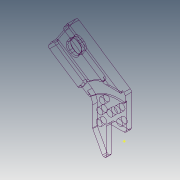
# Autodesk Inventor part: J005046
Saved by Autodesk Inventor 2015 SP1 (Build 190203100, 203)
## iProperties
Created: 2014-10-29
Material: STAINLESS STEEL, 316L
Vendor: HHMI: JFRC - ID&F
Document SubType Name: Sheet Metal
Designer: arnoldj
Density: 8 g/cm^3
Sheet Metal Rule: Default
Description: MBS INLINE REF TAB
Mass: 3.02517 g
Surface Area: 6.77077 cm^2
Volume: 0.378146 cm^3
Project: P-201804
Appearance: Pink
Part Number: J005046
RuleStatus: InUse
AfterDocSave0: file://Part Number Cleaner
DESIGN DEPARTMENT: HHMI: JRC - ID&F
SPECIAL FINISH: NONE
LAB/DEPT: SVOBODA (LAB)
REQUESTING SCIENTIST: SOFRONIEW, NICK
SURFACE ROUGHNESS: 63 Ra
Thickness: 0.050 in
ALTERED ITEM PART NUMBER: N/A
ALTERED ITEM VENDOR: N/A
ALTERED ITEM DESCRIPTION: N/A
Revision Number: A
Autodesk Inventor part; units mm, degrees
note: some values were not read from the file. Chosen so that the rebuilt part matches the saved one: edges of "Fillet8".
ref_plane "YZ Plane" through (0, 0, 0) normal (1, 0, 0) x (0, 1, 0)
sketch "Sketch1" plane through (0, 0, 0) normal (0, 0, 1) x (1, 0, 0)
  line L0 (-4.699, -1.143) -> (-4.699, 6.1251)
  line L1 (4.699, 2.286) -> (4.699, 11.9364)
  line L2 (-4.699, -1.143) -> (-4.699, -1.143) construction
  line L3 (-4.699, -1.143) -> (-1.905, -6.35) construction
  line L4 (-0.889, -6.35) -> (-0.889, 2.286)
  line L5 (4.699, 2.286) -> (-0.889, 2.286)
  line L6 (-0.889, -6.35) -> (-1.905, -6.35)
  line L7 (-1.905, -6.35) -> (-4.699, -1.143)
  line L8 (-4.699, 6.1251) -> (-15.7683, 13.4517)
  line L9 (-15.7683, 13.4517) -> (-10.2307, 21.8181)
  line L10 (-10.2307, 21.8181) -> (4.699, 11.9364)
  line L11 (-15.7683, 13.4517) -> (-28.0607, 13.4517) construction
  line L12 (-12.9995, 17.6349) -> (0, 9.0307) construction
  line L13 (-9.5394, 13.0603) -> (-7.4366, 16.2374)
  line L14 (-7.4366, 16.2374) -> (-10.1053, 18.0038)
  line L15 (-10.1053, 18.0038) -> (-12.2082, 14.8267)
  line L16 (-12.2082, 14.8267) -> (-9.5394, 13.0603)
  line L17 (-9.5394, 13.0603) -> (-10.1053, 18.0038) construction
  line L18 (-7.4366, 16.2374) -> (-12.2082, 14.8267) construction
  point P0 (0, 0)
  point P1 (0, 0)
  point P2 (0, 0)
  point P3 (0, 0)
  point P4 (2.611, -1.214)
  point P5 (-9.8224, 15.532)
  dimension "d102" = 1.016
  dimension "d161" = 123.5
  dimension "d162" = 10.033
  dimension "d168" = 8.636
  dimension "d170" = 5.207
  dimension "d171" = 0.889
  dimension "d172" = 3.5
  dimension "d173" = 3.5
  dimension "d177" = 146.5
  dimension "d180" = 9.0307
  dimension "d181" = 17.6349
  dimension "d182" = 12.9995
  dimension "d209" = 7.31
  dimension "d210" = 2.088
  dimension "d221" = 3.81
  dimension "d232" = 3.2004
  dimension "d233" = 3.81
  constraints: 38 end point, 4 parallel, 4 vertical, 3 horizontal, 3 midpoint, 3 perpendicular, 2 coincident, 2 point on line, 1 collinear
  measures "d102" distance of L4.start L3.end
  measures "d161" angle of L8 L0
  measures "d162" distance of L8.end L9.end
  measures "d168" distance of L4.start L4.end
  measures "d170" distance from line of L0.start L6
  measures "d171" distance from line of L4 point (0, 0)
  measures "d172" distance from line of point (2.611, -1.214) L4
  measures "d173" distance from line of L5 point (2.611, -1.214)
  measures "d177" angle of L8 L11
  measures "d180" distance of L12.end point (0, 0)
  measures "d181" vertical distance of point (0, 0) L12.start
  measures "d182" horizontal distance of point (0, 0) L12.start
  measures "d209" distance from line of point (2.611, -1.214) L0
  measures "d210" distance from line of L1 point (2.611, -1.214)
  measures "d221" distance from line of point (-9.822, 15.532) L9
  measures "d232" distance of L13.end L14.end
  measures "d233" distance of L13.start L13.end
extrude "Plate1" add sketch "Sketch1" along normal blind 1.27 contours L0 L8 L9 L10 L1 L5 L4 L6 L7 | L16 L15 L14 L13
ref_plane "Work Plane1" through (0, 10.16, 0) normal (0, 1, 0) x (-1, 0, 0)
sketch "Sketch7" plane through (0, 0, 0) normal (0, 0, 1) x (1, 0, 0)
  circle A0 centre (0, 4.7752) radius 0.8255
  circle A1 centre (-2.7432, 3.9116) radius 0.8255
  circle A2 centre (2.7432, 3.9116) radius 0.8255
  line L0 (0, 23.2371) -> (0, -13.8278) construction
  circle A3 centre (-2.1082, 6.7056) radius 0.8255
  circle A4 centre (2.1082, 6.7056) radius 0.8255
  circle A5 centre (-2.921, 1.0414) radius 0.8255
  line L1 (-4.699, -1.143) -> (-4.699, 6.1251) projected
  line L2 (-0.889, 2.286) -> (-0.889, -6.35) construction
  line L3 (-1.905, -6.35) -> (-4.699, -1.143) construction
  line L4 (-22.6717, 0) -> (18.6824, 0) projected
  line L5 (4.699, 2.286) -> (-0.889, 2.286) projected
  line L6 (4.699, 11.9364) -> (4.699, 2.286) projected
  point P0 (0, 0)
  dimension "d61" = 1.651
  dimension "d250" = 4.4196
  dimension "d251" = 4.4196
  dimension "d252" = 1.9558
  dimension "d253" = 1.6256
  dimension "d254" = 2.4892
  dimension "d255" = 2.5908
  dimension "d256" = 4.699
  dimension "d257" = 6.8072
  dimension "d258" = 7.4422
  dimension "d259" = 7.62
  dimension "d260" = 1.2446
  dimension "d261" = 1.6256
  constraints: 6 centre point, 5 equal radius, 3 coincident
  measures "d61" diameter of A0
  measures "d250" distance from line of A3.centre L5
  measures "d251" distance from line of L5 point (2.108, 6.706)
  measures "d252" distance from line of L6 A2.centre
  measures "d253" distance from line of point (2.743, 3.912) L5
  measures "d254" distance from line of L5 A0.centre
  measures "d255" distance from line of point (2.108, 6.706) L6
  measures "d256" distance from line of A0.centre L6
  measures "d257" distance from line of A3.centre L6
  measures "d258" distance from line of L6 point (-2.743, 3.912)
  measures "d259" distance from line of A5.centre L6
  measures "d260" distance from line of A5.centre L5
  measures "d261" distance from line of L5 point (-2.743, 3.912)
hole "Hole2" at (-2.7432, 3.9116, 0) at (2.7432, 3.9116, 0) at (0, 4.7752, 0) at (2.1082, 6.7056, 0) at (-2.1082, 6.7056, 0) at (-2.921, 1.0414, 0) direction (0, 0, 1) diameter 1.651 depth 1.27 tip angle 118
sketch "Sketch11" plane through (0, 0, 1.27) normal (0, 0, 1) x (1, 0, 0)
  line L0 (-10.2307, 21.8181) -> (4.699, 11.9364) projected
  line L1 (-4.699, 6.1251) -> (-15.7683, 13.4517) projected
  line L2 (4.699, 11.9364) -> (-10.2307, 21.8181) projected
  line L3 (-15.7683, 13.4517) -> (-10.2307, 21.8181) projected
  circle A0 centre (2.611, -1.214) radius 12.7
  line L4 (-14.4105, 15.5031) -> (-5.6205, 9.6851)
  line L5 (-11.5885, 19.7667) -> (0.242, 11.9364)
  line L6 (-5.6205, 9.6851) -> (-6.9783, 7.6338)
  line L7 (-15.7683, 13.4517) -> (-4.699, 6.1251) projected
  line L8 (-6.9783, 7.6338) -> (-15.7683, 13.4517)
  line L9 (-15.7683, 13.4517) -> (-10.2307, 21.8181)
  line L10 (-10.2307, 21.8181) -> (-15.7683, 13.4517) projected
  line L11 (-10.2307, 21.8181) -> (4.699, 11.9364)
  line L12 (4.699, 2.286) -> (4.699, 11.9364) projected
  line L13 (4.699, 11.9364) -> (0.242, 11.9364)
  line L14 (-7.712, 11.0892) -> (-9.4235, 12.222) projected
  line L15 (-4.9081, 15.3253) -> (-6.6196, 16.4582) projected
  point P0 (0, 0)
  point P1 (-4.9002, 6.2781)
  point P2 (-9.9999, 18.7153)
  point P3 (-12.7869, 14.4284)
  dimension "d183" = 25.4
  dimension "d219" = 2.46
  dimension "d220" = 2.46
  constraints: 14 end point, 4 point on line, 1 centre point, 1 coincident, 1 collinear, 1 horizontal, 1 parallel, 1 perpendicular, 6 other
  measures "d183" diameter of A0
  measures "d219" distance between parallel lines of L8 L4
  measures "d220" distance between parallel lines of L5 L0
extrude "Extrusion3" add sketch "Sketch11" along normal blind 1.27 contours L0 L13 L5 L3 | L4 L6 L1 L3
ref_plane "Work Plane3" through (0, 0, 1.143) normal (0, 0, 1) x (1, 0, 0)
fillet "Fillet4" radius 0.7937 1 edges at (4.699, 2.286, 0.635)
fillet "Fillet7" radius 0.381 3 edges at (-4.699, -1.143, 0.635) (-1.905, -6.35, 0.635) (-0.889, -6.35, 0.635)
fillet "Fillet8" radius 0.7937 1 edges at (4.699, 11.9364, 0.635)
sketch "Sketch12" plane through (0, 0, 1.27) normal (0, 0, 1) x (1, 0, 0)
  arc A0 (4.699, 9.3458) -> (-5.0441, 6.3535) centre (2.611, -1.214) ccw
  line L0 (-6.9783, 7.6338) -> (-5.0441, 6.3535)
  line L1 (4.699, 9.3458) -> (4.699, 11.5099)
  arc A1 (-0.1461, 12.1631) -> (-5.6205, 9.6851) centre (2.611, -1.214) ccw
  line L2 (-5.6205, 9.6851) -> (-6.9783, 7.6338)
  line L3 (-6.9783, 7.6338) -> (-5.6205, 9.6851) projected
  arc A2 (4.0458, 12.3687) -> (-0.1461, 12.1631) centre (2.611, -1.214) ccw
  line L4 (4.3433, 12.1718) -> (-10.2307, 21.8181) projected
  arc A3 (4.5747, 11.9364) -> (4.3433, 12.1718) centre (3.9052, 11.5099) ccw projected
  arc A4 (4.699, 11.5099) -> (4.3433, 12.1718) centre (3.9052, 11.5099) ccw projected
  arc A5 (4.699, 11.5099) -> (4.3433, 12.1718) centre (3.9052, 11.5099) ccw
  line L5 (4.0458, 12.3687) -> (4.3433, 12.1718)
  line L6 (4.3433, 12.1718) -> (-10.2307, 21.8181) projected
  line L7 (-4.699, 6.1251) -> (-6.9783, 7.6338) projected
  point P0 (0, 0)
  point P1 (0.242, 11.9364)
  point P2 (3.9052, 11.4901)
  point P3 (-9.6044, 21.3838)
  point P4 (-10.2307, 21.8181)
  constraints: 8 end point, 8 point on circle, 4 centre point, 3 coincident, 1 collinear, 1 point on line, 1 vertical, 3 other
extrude "Extrusion5" add sketch "Sketch12" along normal blind 0.4826
chamfer "Chamfer4" distance 0.381 angle 45 2 edges at (-6.2994, 8.6594, 2.54) (2.4083, 11.9364, 2.54)
fillet "Fillet12" radius 0.635 1 edges at (-6.9783, 7.6338, 1.9558)
fillet "Fillet13" radius 0.635 3 edges at (0.242, 11.9364, 1.9558) (4.699, 9.3458, 1.5113) (-5.0441, 6.3535, 1.5113)
sketch "Sketch9" plane through (0, 0, 0) normal (0, 0, 1) x (1, 0, 0)
  point P0 (0, 0)
sketch "Sketch10" plane through (0, 0, 0) normal (0, 0, 1) x (1, 0, 0)
  circle A0 centre (2.6461, -1.2506) radius 3.5
  point P0 (0, 0)
  dimension "d150" = 7
  constraints: 1 centre point
  measures "d150" diameter of A0
ref_plane "Work Plane5" through (-10.0977, 15.7143, 1.016) normal (0.551937, 0.8338858, 0) x (0.8338858, -0.551937, 0)
ref_plane "Work Plane6" through (-10.1729, 15.0025, 0.254) normal (-0.8338858, 0.551937, 0) x (0, 0, 1)
sketch "Sketch3" plane through (0, 0, 1.27) normal (0, 0, 1) x (1, 0, 0)
  line L0 (-16.764, 14.16) -> (4.445, 14.16)
  line L1 (-4.445, 6.16) -> (-16.764, 6.16)
  line L2 (-6.35, 14.16) -> (-6.35, 6.16)
  line L3 (0, 17.9421) -> (0, -8.5328)
  line L4 (12.7747, 8.2785) -> (4.445, 8.2785)
  point P0 (0, 0)
  point P1 (-5.2531, 14.0148)
  point P2 (4.445, 14.16)
  dimension "d15" = 6.35
  constraints: 8 end point, 1 perpendicular, 1 point on line, 4 other
  measures "d15" distance between parallel lines of L3 L2
fillet "Fillet14" radius 3.175 1 edges at (-4.699, 6.1251, 0.635)
fillet "Fillet15" radius 1.016 1 edges at (-0.889, 2.286, 0.635)
fillet "Fillet16" radius 0.254 1 edges at (4.5747, 11.9364, 1.9558)
fillet "Fillet17" radius 0.635 2 edges at (-5.6205, 9.6851, 1.5113) (-0.1114, 12.1702, 1.5113)
fillet "Fillet18" radius 0.635 1 edges at (-5.5218, 9.8342, 1.9558)
sketch "Sketch15" plane through (0, 0, 0) normal (0, 0, 1) x (1, 0, 0)
  point P0 (0, 0)
extrude "Extrusion7" cut sketch "Sketch1" along normal up to next contours L16 L15 L14 L13
fillet "Fillet19" radius 1.27 4 edges at (-7.4366, 16.2374, 0.635) (-9.5394, 13.0603, 0.635) (-12.2082, 14.8267, 0.635) (-10.1053, 18.0038, 0.635)
chamfer "Chamfer6" distance 0.254 angle 45 16 edges at (-8.488, 14.6488, 1.27) (-9.6443, 13.5758, 1.27) (-10.8738, 13.9435, 1.27) (-11.6927, 14.9316, 1.27) (-11.1568, 16.4152, 1.27) (-10.0004, 17.4883, 1.27) (-8.7709, 17.1206, 1.27) (-7.952, 16.1325, 1.27) (-7.952, 16.1325, 0) (-8.488, 14.6488, 0) (-9.6443, 13.5758, 0) (-10.8738, 13.9435, 0) (-11.6927, 14.9316, 0) (-11.1568, 16.4152, 0) (-10.0004, 17.4883, 0) (-8.7709, 17.1206, 0)
fillet "Fillet20" radius 0.635 4 edges at (-11.5885, 19.7667, 1.905) (-14.4105, 15.5031, 1.905) (-15.7683, 13.4517, 1.27) (-10.2307, 21.8181, 1.27)
equation "\"d71\" = Thickness"
equation "\"BendRadius\" = Thickness"
equation "\"BendReliefWidth\" = Thickness"
equation "\"BendReliefDepth\" = 0.5 * Thickness"
equation "\"CornerReliefSize\" = 4 * Thickness"
equation "\"MinimumRemnant\" = 2 * Thickness"
equation "\"TransitionRadius\" = BendRadius"
equation "\"JacobiRadiusSize\" = BendRadius"
equation "\"GapSize\" = Thickness"
equation "\"d6\" = BendRadius"
equation "\"Thickness\" = 1.27"
body "Solid1"
